Autodesk Inventor part; units mm, degrees
(part 2 of 3)
  spline S225 degree 2 poles (-23.0863, -3.6473) (-22.622, -3.6473) (-22.0662, -4.2796) (-22.0662, -4.8551) knots 0 0 0 1 2 2 2
  spline S226 degree 2 poles (-22.4639, -4.8551) (-22.4639, -4.4105) (-22.7874, -3.9782) (-23.0863, -3.9782) knots 0 0 0 1 2 2 2
  spline S227 degree 2 poles (-23.0863, -3.9782) (-23.3852, -3.9782) (-23.7112, -4.4105) (-23.7112, -4.8551) knots 0 0 0 1 2 2 2
  spline S228 degree 2 poles (-23.7112, -4.8551) (-23.7112, -5.2874) (-23.3852, -5.732) (-23.0863, -5.732) knots 0 0 0 1 2 2 2
  spline S229 degree 2 poles (-23.0863, -5.732) (-22.7899, -5.732) (-22.4639, -5.2948) (-22.4639, -4.8551) knots 0 0 0 1 2 2 2
  line L249 (-1.1, 56.7348) -> (1.5874, 56.7348)
  line L250 (1.5874, 56.7348) -> (1.5874, 57.7574)
  line L251 (1.5874, 57.7574) -> (1.948, 57.7574)
  line L252 (1.948, 57.7574) -> (1.948, 55.3071)
  line L253 (1.948, 55.3071) -> (1.5874, 55.3071)
  line L254 (1.5874, 55.3071) -> (1.5874, 56.3297)
  line L255 (1.5874, 56.3297) -> (-1.1, 56.3297)
  line L256 (-1.1, 56.3297) -> (-1.1, 56.7348)
  spline S230 degree 2 poles (0.0436, 53.1483) (-0.5344, 53.1483) (-1.1642, 53.7041) (-1.1642, 54.1685) knots 0 0 0 1 2 2 2
  spline S231 degree 2 poles (-1.1642, 54.1685) (-1.1642, 54.6452) (-0.5146, 55.191) (0.0436, 55.191) knots 0 0 0 1 2 2 2
  spline S232 degree 2 poles (0.0436, 55.191) (0.6167, 55.191) (1.2515, 54.6279) (1.2515, 54.1685) knots 0 0 0 1 2 2 2
  spline S233 degree 2 poles (1.2515, 54.1685) (1.2515, 53.7041) (0.6191, 53.1483) (0.0436, 53.1483) knots 0 0 0 1 2 2 2
  spline S234 degree 2 poles (0.0436, 53.546) (0.4882, 53.546) (0.9205, 53.8696) (0.9205, 54.1685) knots 0 0 0 1 2 2 2
  spline S235 degree 2 poles (0.9205, 54.1685) (0.9205, 54.4673) (0.4882, 54.7934) (0.0436, 54.7934) knots 0 0 0 1 2 2 2
  spline S236 degree 2 poles (0.0436, 54.7934) (-0.3886, 54.7934) (-0.8332, 54.4673) (-0.8332, 54.1685) knots 0 0 0 1 2 2 2
  spline S237 degree 2 poles (-0.8332, 54.1685) (-0.8332, 53.8721) (-0.396, 53.546) (0.0436, 53.546) knots 0 0 0 1 2 2 2
  line L257 (0.7747, 51.5404) -> (0.7747, 51.5601)
  spline S238 degree 2 poles (0.7747, 51.5601) (0.7871, 51.6046) (0.792, 51.7009) (0.792, 51.7676) knots 0 0 0 1 2 2 2
  spline S239 degree 2 poles (0.792, 51.7676) (0.792, 51.9232) (0.6562, 52.2295) (0.5228, 52.3678) knots 0 0 0 1 2 2 2
  line L258 (0.5228, 52.3678) -> (-1.1, 52.3678)
  line L259 (-1.1, 52.3678) -> (-1.1, 52.7531)
  line L260 (-1.1, 52.7531) -> (1.1872, 52.7531)
  line L261 (1.1872, 52.7531) -> (1.1872, 52.3678)
  line L262 (1.1872, 52.3678) -> (0.8464, 52.3678)
  spline S240 degree 2 poles (0.8464, 52.3678) (1.0341, 52.1579) (1.1872, 51.8442) (1.1872, 51.696) knots 0 0 0 1 2 2 2
  spline S241 degree 2 poles (1.1872, 51.696) (1.1872, 51.6367) (1.1823, 51.5774) (1.1749, 51.5404) knots 0 0 0 1 2 2 2
  line L263 (1.1749, 51.5404) -> (0.7747, 51.5404)
  line L264 (1.948, 47.6921) -> (-1.1, 48.7418)
  line L265 (-1.1, 48.7418) -> (-1.1, 49.179)
  line L266 (-1.1, 49.179) -> (1.948, 50.2288)
  line L267 (1.948, 50.2288) -> (1.948, 49.7941)
  line L268 (1.948, 49.7941) -> (-0.5838, 48.9493)
  line L269 (-0.5838, 48.9493) -> (1.948, 48.1046)
  line L270 (1.948, 48.1046) -> (1.948, 47.6921)
  spline S242 degree 2 poles (-1.1519, 46.4373) (-1.1519, 46.9856) (-0.5368, 47.5883) (0.0313, 47.5883) knots 0 0 0 1 2 2 2
  spline S243 degree 2 poles (0.0313, 47.5883) (0.5895, 47.5883) (1.2515, 47.0029) (1.2515, 46.5312) knots 0 0 0 1 2 2 2
  spline S244 degree 2 poles (1.2515, 46.5312) (1.2515, 46.3187) (1.128, 45.9902) (0.997, 45.8692) knots 0 0 0 1 2 2 2
  spline S245 degree 2 poles (0.997, 45.8692) (0.8661, 45.7457) (0.4882, 45.6148) (0.2141, 45.6148) knots 0 0 0 1 2 2 2
  line L271 (0.2141, 45.6148) -> (0.0041, 45.6148)
  line L272 (0.0041, 45.6148) -> (0.0041, 47.1981)
  spline S246 degree 2 poles (0.0041, 47.1981) (-0.3936, 47.1981) (-0.8159, 46.7979) (-0.8159, 46.4422) knots 0 0 0 1 2 2 2
  spline S247 degree 2 poles (-0.8159, 46.4422) (-0.8159, 46.3163) (-0.7591, 46.0717) (-0.7147, 45.9729) knots 0 0 0 1 2 2 2
  spline S248 degree 2 poles (-0.7147, 45.9729) (-0.6653, 45.8692) (-0.5788, 45.7259) (-0.5393, 45.679) knots 0 0 0 1 2 2 2
  line L273 (-0.5393, 45.679) -> (-0.5393, 45.6568)
  line L274 (-0.5393, 45.6568) -> (-0.9592, 45.6568)
  spline S249 degree 2 poles (-0.9592, 45.6568) (-0.9864, 45.7235) (-1.0654, 45.926) (-1.0876, 46.0051) knots 0 0 0 1 2 2 2
  spline S250 degree 2 poles (-1.0876, 46.0051) (-1.1198, 46.1162) (-1.1519, 46.299) (-1.1519, 46.4373) knots 0 0 0 1 2 2 2
  spline S251 degree 2 poles (0.298, 45.9902) (0.4536, 45.9952) (0.6809, 46.0594) (0.7575, 46.1211) knots 0 0 0 1 2 2 2
  spline S252 degree 2 poles (0.7575, 46.1211) (0.8439, 46.1878) (0.9353, 46.3978) (0.9353, 46.5534) knots 0 0 0 1 2 2 2
  spline S253 degree 2 poles (0.9353, 46.5534) (0.9353, 46.7065) (0.8439, 46.9214) (0.755, 47.0103) knots 0 0 0 1 2 2 2
  spline S254 degree 2 poles (0.755, 47.0103) (0.6636, 47.0968) (0.4438, 47.1857) (0.298, 47.1981) knots 0 0 0 1 2 2 2
  line L275 (0.298, 47.1981) -> (0.298, 45.9902)
  line L276 (0.7747, 44.0117) -> (0.7747, 44.0315)
  spline S255 degree 2 poles (0.7747, 44.0315) (0.7871, 44.076) (0.792, 44.1723) (0.792, 44.239) knots 0 0 0 1 2 2 2
  spline S256 degree 2 poles (0.792, 44.239) (0.792, 44.3946) (0.6562, 44.7009) (0.5228, 44.8392) knots 0 0 0 1 2 2 2
  line L277 (0.5228, 44.8392) -> (-1.1, 44.8392)
  line L278 (-1.1, 44.8392) -> (-1.1, 45.2245)
  line L279 (-1.1, 45.2245) -> (1.1872, 45.2245)
  line L280 (1.1872, 45.2245) -> (1.1872, 44.8392)
  line L281 (1.1872, 44.8392) -> (0.8464, 44.8392)
  spline S257 degree 2 poles (0.8464, 44.8392) (1.0341, 44.6293) (1.1872, 44.3156) (1.1872, 44.1674) knots 0 0 0 1 2 2 2
  spline S258 degree 2 poles (1.1872, 44.1674) (1.1872, 44.1081) (1.1823, 44.0488) (1.1749, 44.0117) knots 0 0 0 1 2 2 2
  line L282 (1.1749, 44.0117) -> (0.7747, 44.0117)
  spline S259 degree 2 poles (-1.4656, 43.6314) (-1.4829, 43.5918) (-1.5372, 43.4412) (-1.5594, 43.3448) knots 0 0 0 1 2 2 2
  spline S260 degree 2 poles (-1.5594, 43.3448) (-1.5866, 43.2386) (-1.6187, 43.0583) (-1.6187, 42.9521) knots 0 0 0 1 2 2 2
  spline S261 degree 2 poles (-1.6187, 42.9521) (-1.6187, 42.7743) (-1.5248, 42.5273) (-1.4409, 42.4581) knots 0 0 0 1 2 2 2
  spline S262 degree 2 poles (-1.4409, 42.4581) (-1.3569, 42.3914) (-1.137, 42.3395) (-0.9963, 42.3395) knots 0 0 0 1 2 2 2
  line L283 (-0.9963, 42.3395) -> (-0.7962, 42.3395)
  spline S263 degree 2 poles (-0.7962, 42.3395) (-0.932, 42.4952) (-1.0605, 42.794) (-1.0605, 43.0188) knots 0 0 0 1 2 2 2
  spline S264 degree 2 poles (-1.0605, 43.0188) (-1.0605, 43.4091) (-0.48, 43.871) (0.0658, 43.871) knots 0 0 0 1 2 2 2
  spline S265 degree 2 poles (0.0658, 43.871) (0.3499, 43.871) (0.7896, 43.7104) (0.9452, 43.577) knots 0 0 0 1 2 2 2
  spline S266 degree 2 poles (0.9452, 43.577) (1.0909, 43.4486) (1.2515, 43.0954) (1.2515, 42.9077) knots 0 0 0 1 2 2 2
  spline S267 degree 2 poles (1.2515, 42.9077) (1.2515, 42.7298) (1.1675, 42.4705) (1.0909, 42.3395) knots 0 0 0 1 2 2 2
  line L284 (1.0909, 42.3395) -> (1.1872, 42.3173)
  line L285 (1.1872, 42.3173) -> (1.1872, 41.9542)
  line L286 (1.1872, 41.9542) -> (-0.8382, 41.9542)
  spline S268 degree 2 poles (-0.8382, 41.9542) (-1.4211, 41.9542) (-1.9645, 42.4606) (-1.9645, 42.9818) knots 0 0 0 1 2 2 2
  spline S269 degree 2 poles (-1.9645, 42.9818) (-1.9645, 43.1497) (-1.9102, 43.5005) (-1.8657, 43.6511) knots 0 0 0 1 2 2 2
  line L287 (-1.8657, 43.6511) -> (-1.4656, 43.6511)
  line L288 (-1.4656, 43.6511) -> (-1.4656, 43.6314)
  line L289 (-0.48, 42.3395) -> (0.7772, 42.3395)
  spline S270 degree 2 poles (0.7772, 42.3395) (0.8464, 42.4828) (0.9057, 42.7249) (0.9057, 42.8459) knots 0 0 0 1 2 2 2
  spline S271 degree 2 poles (0.9057, 42.8459) (0.9057, 43.1374) (0.4759, 43.4733) (0.0733, 43.4733) knots 0 0 0 1 2 2 2
  spline S272 degree 2 poles (0.0733, 43.4733) (-0.3071, 43.4733) (-0.7048, 43.2189) (-0.7048, 42.9324) knots 0 0 0 1 2 2 2
  spline S273 degree 2 poles (-0.7048, 42.9324) (-0.7048, 42.7817) (-0.5862, 42.4655) (-0.48, 42.3395) knots 0 0 0 1 2 2 2
  spline S274 degree 2 poles (-0.8579, 40.1215) (-0.8925, 40.1684) (-1.016, 40.3265) (-1.0531, 40.4006) knots 0 0 0 1 2 2 2
  spline S275 degree 2 poles (-1.0531, 40.4006) (-1.1074, 40.5019) (-1.1642, 40.692) (-1.1642, 40.8649) knots 0 0 0 1 2 2 2
  spline S276 degree 2 poles (-1.1642, 40.8649) (-1.1642, 41.0057) (-1.058, 41.2601) (-0.9617, 41.3565) knots 0 0 0 1 2 2 2
  spline S277 degree 2 poles (-0.9617, 41.3565) (-0.8678, 41.4479) (-0.5912, 41.559) (-0.438, 41.559) knots 0 0 0 1 2 2 2
  spline S278 degree 2 poles (-0.438, 41.559) (-0.2009, 41.559) (0.135, 41.3589) (0.2313, 41.1416) knots 0 0 0 1 2 2 2
  spline S279 degree 2 poles (0.2313, 41.1416) (0.3203, 40.9489) (0.387, 40.4253) (0.4042, 40.1215) knots 0 0 0 1 2 2 2
  line L290 (0.4042, 40.1215) -> (0.4783, 40.1215)
  spline S280 degree 2 poles (0.4783, 40.1215) (0.6117, 40.1215) (0.7772, 40.203) (0.8241, 40.2771) knots 0 0 0 1 2 2 2
  spline S281 degree 2 poles (0.8241, 40.2771) (0.8711, 40.3512) (0.9007, 40.5636) (0.9007, 40.6772) knots 0 0 0 1 2 2 2
  spline S282 degree 2 poles (0.9007, 40.6772) (0.9007, 40.8106) (0.8217, 41.1712) (0.7451, 41.3515) knots 0 0 0 1 2 2 2
  line L291 (0.7451, 41.3515) -> (0.7451, 41.3738)
  line L292 (0.7451, 41.3738) -> (1.1378, 41.3738)
  spline S283 degree 2 poles (1.1378, 41.3738) (1.1675, 41.2676) (1.2416, 40.8699) (1.2416, 40.6748) knots 0 0 0 1 2 2 2
  spline S284 degree 2 poles (1.2416, 40.6748) (1.2416, 40.4376) (1.1675, 40.1141) (1.0711, 39.9856) knots 0 0 0 1 2 2 2
  spline S285 degree 2 poles (1.0711, 39.9856) (0.9773, 39.8596) (0.6784, 39.7361) (0.4635, 39.7361) knots 0 0 0 1 2 2 2
  line L293 (0.4635, 39.7361) -> (-1.1, 39.7361)
  line L294 (-1.1, 39.7361) -> (-1.1, 40.1215)
  line L295 (-1.1, 40.1215) -> (-0.8579, 40.1215)
  line L296 (-0.5368, 40.1215) -> (0.098, 40.1215)
  spline S286 degree 2 poles (0.098, 40.1215) (0.0856, 40.2598) (0.0436, 40.6772) (0.0041, 40.8081) knots 0 0 0 1 2 2 2
  spline S287 degree 2 poles (0.0041, 40.8081) (-0.0428, 40.9613) (-0.238, 41.1613) (-0.4109, 41.1613) knots 0 0 0 1 2 2 2
  spline S288 degree 2 poles (-0.4109, 41.1613) (-0.6085, 41.1613) (-0.8085, 40.939) (-0.8085, 40.7266) knots 0 0 0 1 2 2 2
  spline S289 degree 2 poles (-0.8085, 40.7266) (-0.8085, 40.5463) (-0.6529, 40.2499) (-0.5368, 40.1215) knots 0 0 0 1 2 2 2
  spline S290 degree 2 poles (-1.1445, 38.5036) (-1.1445, 38.8173) (-0.7863, 39.1705) (-0.3985, 39.1705) knots 0 0 0 1 2 2 2
  line L297 (-0.3985, 39.1705) -> (0.8686, 39.1705)
  line L298 (0.8686, 39.1705) -> (0.8686, 39.4299)
  line L299 (0.8686, 39.4299) -> (1.1872, 39.4299)
  line L300 (1.1872, 39.4299) -> (1.1872, 39.1705)
  line L301 (1.1872, 39.1705) -> (1.8443, 39.1705)
  line L302 (1.8443, 39.1705) -> (1.8443, 38.7852)
  line L303 (1.8443, 38.7852) -> (1.1872, 38.7852)
  line L304 (1.1872, 38.7852) -> (1.1872, 38.0763)
  line L305 (1.1872, 38.0763) -> (0.8686, 38.0763)
  line L306 (0.8686, 38.0763) -> (0.8686, 38.7852)
  line L307 (0.8686, 38.7852) -> (-0.2207, 38.7852)
  spline S291 degree 2 poles (-0.2207, 38.7852) (-0.3936, 38.7852) (-0.5838, 38.7728) (-0.6653, 38.7309) knots 0 0 0 1 2 2 2
  spline S292 degree 2 poles (-0.6653, 38.7309) (-0.7369, 38.6963) (-0.8085, 38.5407) (-0.8085, 38.4073) knots 0 0 0 1 2 2 2
  spline S293 degree 2 poles (-0.8085, 38.4073) (-0.8085, 38.3134) (-0.7517, 38.138) (-0.7344, 38.0985) knots 0 0 0 1 2 2 2
  line L308 (-0.7344, 38.0985) -> (-0.7344, 38.0763)
  line L309 (-0.7344, 38.0763) -> (-1.0802, 38.0763)
  spline S294 degree 2 poles (-1.0802, 38.0763) (-1.1099, 38.185) (-1.1445, 38.4073) (-1.1445, 38.5036) knots 0 0 0 1 2 2 2
  spline S295 degree 2 poles (-0.8579, 36.5177) (-0.8925, 36.5646) (-1.016, 36.7227) (-1.0531, 36.7968) knots 0 0 0 1 2 2 2
  spline S296 degree 2 poles (-1.0531, 36.7968) (-1.1074, 36.8981) (-1.1642, 37.0883) (-1.1642, 37.2612) knots 0 0 0 1 2 2 2
  spline S297 degree 2 poles (-1.1642, 37.2612) (-1.1642, 37.402) (-1.058, 37.6564) (-0.9617, 37.7527) knots 0 0 0 1 2 2 2
  spline S298 degree 2 poles (-0.9617, 37.7527) (-0.8678, 37.8441) (-0.5912, 37.9553) (-0.438, 37.9553) knots 0 0 0 1 2 2 2
  spline S299 degree 2 poles (-0.438, 37.9553) (-0.2009, 37.9553) (0.135, 37.7552) (0.2313, 37.5378) knots 0 0 0 1 2 2 2
  spline S300 degree 2 poles (0.2313, 37.5378) (0.3203, 37.3452) (0.387, 36.8215) (0.4042, 36.5177) knots 0 0 0 1 2 2 2
  line L310 (0.4042, 36.5177) -> (0.4783, 36.5177)
  spline S301 degree 2 poles (0.4783, 36.5177) (0.6117, 36.5177) (0.7772, 36.5992) (0.8241, 36.6733) knots 0 0 0 1 2 2 2
  spline S302 degree 2 poles (0.8241, 36.6733) (0.8711, 36.7474) (0.9007, 36.9599) (0.9007, 37.0735) knots 0 0 0 1 2 2 2
  spline S303 degree 2 poles (0.9007, 37.0735) (0.9007, 37.2069) (0.8217, 37.5675) (0.7451, 37.7478) knots 0 0 0 1 2 2 2
  line L311 (0.7451, 37.7478) -> (0.7451, 37.77)
  line L312 (0.7451, 37.77) -> (1.1378, 37.77)
  spline S304 degree 2 poles (1.1378, 37.77) (1.1675, 37.6638) (1.2416, 37.2661) (1.2416, 37.071) knots 0 0 0 1 2 2 2
  spline S305 degree 2 poles (1.2416, 37.071) (1.2416, 36.8339) (1.1675, 36.5103) (1.0711, 36.3819) knots 0 0 0 1 2 2 2
  spline S306 degree 2 poles (1.0711, 36.3819) (0.9773, 36.2559) (0.6784, 36.1324) (0.4635, 36.1324) knots 0 0 0 1 2 2 2
  line L313 (0.4635, 36.1324) -> (-1.1, 36.1324)
  line L314 (-1.1, 36.1324) -> (-1.1, 36.5177)
  line L315 (-1.1, 36.5177) -> (-0.8579, 36.5177)
  line L316 (-0.5368, 36.5177) -> (0.098, 36.5177)
  spline S307 degree 2 poles (0.098, 36.5177) (0.0856, 36.656) (0.0436, 37.0735) (0.0041, 37.2044) knots 0 0 0 1 2 2 2
  spline S308 degree 2 poles (0.0041, 37.2044) (-0.0428, 37.3575) (-0.238, 37.5576) (-0.4109, 37.5576) knots 0 0 0 1 2 2 2
  spline S309 degree 2 poles (-0.4109, 37.5576) (-0.6085, 37.5576) (-0.8085, 37.3353) (-0.8085, 37.1229) knots 0 0 0 1 2 2 2
  spline S310 degree 2 poles (-0.8085, 37.1229) (-0.8085, 36.9426) (-0.6529, 36.6462) (-0.5368, 36.5177) knots 0 0 0 1 2 2 2
  spline S311 degree 2 poles (28.9328, 4.0036) (28.6019, 4.0036) (28.1375, 4.1419) (27.9325, 4.2407) knots 0 0 0 1 2 2 2
  line L317 (27.9325, 4.2407) -> (27.9325, 4.7495)
  line L318 (27.9325, 4.7495) -> (27.9621, 4.7495)
  spline S312 degree 2 poles (27.9621, 4.7495) (28.1622, 4.5618) (28.6686, 4.3543) (28.9032, 4.3543) knots 0 0 0 1 2 2 2
  spline S313 degree 2 poles (28.9032, 4.3543) (29.2391, 4.3543) (29.5825, 4.6335) (29.5825, 4.8632) knots 0 0 0 1 2 2 2
  spline S314 degree 2 poles (29.5825, 4.8632) (29.5825, 5.046) (29.4022, 5.2732) (29.207, 5.33) knots 0 0 0 1 2 2 2
  spline S315 degree 2 poles (29.207, 5.33) (29.0662, 5.3695) (28.8316, 5.4239) (28.6562, 5.4683) knots 0 0 0 1 2 2 2
  spline S316 degree 2 poles (28.6562, 5.4683) (28.4981, 5.5103) (28.2487, 5.6363) (28.1523, 5.7376) knots 0 0 0 1 2 2 2
  spline S317 degree 2 poles (28.1523, 5.7376) (28.0585, 5.8388) (27.9547, 6.1105) (27.9547, 6.2884) knots 0 0 0 1 2 2 2
  spline S318 degree 2 poles (27.9547, 6.2884) (27.9547, 6.6589) (28.5327, 7.1603) (28.9798, 7.1603) knots 0 0 0 1 2 2 2
  spline S319 degree 2 poles (28.9798, 7.1603) (29.2367, 7.1603) (29.6911, 7.059) (29.8863, 6.9627) knots 0 0 0 1 2 2 2
  line L319 (29.8863, 6.9627) -> (29.8863, 6.4786)
  line L320 (29.8863, 6.4786) -> (29.8566, 6.4786)
  spline S320 degree 2 poles (29.8566, 6.4786) (29.7109, 6.6119) (29.2564, 6.8095) (29.0069, 6.8095) knots 0 0 0 1 2 2 2
  spline S321 degree 2 poles (29.0069, 6.8095) (28.7254, 6.8095) (28.3771, 6.5453) (28.3771, 6.3304) knots 0 0 0 1 2 2 2
  spline S322 degree 2 poles (28.3771, 6.3304) (28.3771, 6.1377) (28.5821, 5.908) (28.7748, 5.8561) knots 0 0 0 1 2 2 2
  spline S323 degree 2 poles (28.7748, 5.8561) (28.9032, 5.8215) (29.2762, 5.7326) (29.3997, 5.6956) knots 0 0 0 1 2 2 2
  spline S324 degree 2 poles (29.3997, 5.6956) (29.7134, 5.5992) (30.0048, 5.2114) (30.0048, 4.9274) knots 0 0 0 1 2 2 2
  spline S325 degree 2 poles (30.0048, 4.9274) (30.0048, 4.7471) (29.8591, 4.4013) (29.7282, 4.2802) knots 0 0 0 1 2 2 2
  spline S326 degree 2 poles (29.7282, 4.2802) (29.5825, 4.1469) (29.212, 4.0036) (28.9328, 4.0036) knots 0 0 0 1 2 2 2
  spline S327 degree 2 poles (32.2674, 5.2016) (32.2674, 4.6236) (31.7116, 3.9937) (31.2473, 3.9937) knots 0 0 0 1 2 2 2
  spline S328 degree 2 poles (31.2473, 3.9937) (30.7705, 3.9937) (30.2247, 4.6433) (30.2247, 5.2016) knots 0 0 0 1 2 2 2
  spline S329 degree 2 poles (30.2247, 5.2016) (30.2247, 5.7746) (30.7878, 6.4094) (31.2473, 6.4094) knots 0 0 0 1 2 2 2
  spline S330 degree 2 poles (31.2473, 6.4094) (31.7116, 6.4094) (32.2674, 5.7771) (32.2674, 5.2016) knots 0 0 0 1 2 2 2
  spline S331 degree 2 poles (31.8697, 5.2016) (31.8697, 5.6462) (31.5461, 6.0784) (31.2473, 6.0784) knots 0 0 0 1 2 2 2
  spline S332 degree 2 poles (31.2473, 6.0784) (30.9484, 6.0784) (30.6223, 5.6462) (30.6223, 5.2016) knots 0 0 0 1 2 2 2
  spline S333 degree 2 poles (30.6223, 5.2016) (30.6223, 4.7693) (30.9484, 4.3247) (31.2473, 4.3247) knots 0 0 0 1 2 2 2
  spline S334 degree 2 poles (31.2473, 4.3247) (31.5437, 4.3247) (31.8697, 4.7619) (31.8697, 5.2016) knots 0 0 0 1 2 2 2
  spline S335 degree 2 poles (33.5715, 4.0061) (33.3344, 4.0061) (32.9417, 4.1518) (32.8009, 4.3) knots 0 0 0 1 2 2 2
  spline S336 degree 2 poles (32.8009, 4.3) (32.6601, 4.4457) (32.5045, 4.8953) (32.5045, 5.1966) knots 0 0 0 1 2 2 2
  spline S337 degree 2 poles (32.5045, 5.1966) (32.5045, 5.498) (32.665, 5.9376) (32.8009, 6.0858) knots 0 0 0 1 2 2 2
  spline S338 degree 2 poles (32.8009, 6.0858) (32.9367, 6.2365) (33.3394, 6.397) (33.5715, 6.397) knots 0 0 0 1 2 2 2
  spline S339 degree 2 poles (33.5715, 6.397) (33.7593, 6.397) (34.11, 6.2908) (34.2459, 6.2217) knots 0 0 0 1 2 2 2
  line L321 (34.2459, 6.2217) -> (34.2459, 5.7894)
  line L322 (34.2459, 5.7894) -> (34.2236, 5.7894)
  spline S340 degree 2 poles (34.2236, 5.7894) (34.1816, 5.824) (34.0532, 5.9129) (33.9618, 5.9599) knots 0 0 0 1 2 2 2
  spline S341 degree 2 poles (33.9618, 5.9599) (33.8803, 5.9994) (33.6629, 6.0611) (33.5641, 6.0611) knots 0 0 0 1 2 2 2
  spline S342 degree 2 poles (33.5641, 6.0611) (33.2653, 6.0611) (32.9022, 5.6091) (32.9022, 5.1966) knots 0 0 0 1 2 2 2
  spline S343 degree 2 poles (32.9022, 5.1966) (32.9022, 4.794) (33.2529, 4.342) (33.5641, 4.342) knots 0 0 0 1 2 2 2
  spline S344 degree 2 poles (33.5641, 4.342) (33.7519, 4.342) (34.0927, 4.4976) (34.2236, 4.6186) knots 0 0 0 1 2 2 2
  line L323 (34.2236, 4.6186) -> (34.2459, 4.6186)
  line L324 (34.2459, 4.6186) -> (34.2459, 4.1864)
  spline S345 degree 2 poles (34.2459, 4.1864) (34.189, 4.1592) (34.0161, 4.0826) (33.947, 4.0654) knots 0 0 0 1 2 2 2
  spline S346 degree 2 poles (33.947, 4.0654) (33.8482, 4.0357) (33.6926, 4.0061) (33.5715, 4.0061) knots 0 0 0 1 2 2 2
  spline S347 degree 2 poles (35.5056, 4.0061) (35.2684, 4.0061) (34.8757, 4.1518) (34.7349, 4.3) knots 0 0 0 1 2 2 2
  spline S348 degree 2 poles (34.7349, 4.3) (34.5941, 4.4457) (34.4385, 4.8953) (34.4385, 5.1966) knots 0 0 0 1 2 2 2
  spline S349 degree 2 poles (34.4385, 5.1966) (34.4385, 5.498) (34.5991, 5.9376) (34.7349, 6.0858) knots 0 0 0 1 2 2 2
  spline S350 degree 2 poles (34.7349, 6.0858) (34.8708, 6.2365) (35.2734, 6.397) (35.5056, 6.397) knots 0 0 0 1 2 2 2
  spline S351 degree 2 poles (35.5056, 6.397) (35.6933, 6.397) (36.044, 6.2908) (36.1799, 6.2217) knots 0 0 0 1 2 2 2
  line L325 (36.1799, 6.2217) -> (36.1799, 5.7894)
  line L326 (36.1799, 5.7894) -> (36.1576, 5.7894)
  spline S352 degree 2 poles (36.1576, 5.7894) (36.1157, 5.824) (35.9872, 5.9129) (35.8958, 5.9599) knots 0 0 0 1 2 2 2
  spline S353 degree 2 poles (35.8958, 5.9599) (35.8143, 5.9994) (35.597, 6.0611) (35.4982, 6.0611) knots 0 0 0 1 2 2 2
  spline S354 degree 2 poles (35.4982, 6.0611) (35.1993, 6.0611) (34.8362, 5.6091) (34.8362, 5.1966) knots 0 0 0 1 2 2 2
  spline S355 degree 2 poles (34.8362, 5.1966) (34.8362, 4.794) (35.1869, 4.342) (35.4982, 4.342) knots 0 0 0 1 2 2 2
  spline S356 degree 2 poles (35.4982, 4.342) (35.6859, 4.342) (36.0267, 4.4976) (36.1576, 4.6186) knots 0 0 0 1 2 2 2
  line L327 (36.1576, 4.6186) -> (36.1799, 4.6186)
  line L328 (36.1799, 4.6186) -> (36.1799, 4.1864)
  spline S357 degree 2 poles (36.1799, 4.1864) (36.1231, 4.1592) (35.9502, 4.0826) (35.881, 4.0654) knots 0 0 0 1 2 2 2
  spline S358 degree 2 poles (35.881, 4.0654) (35.7822, 4.0357) (35.6266, 4.0061) (35.5056, 4.0061) knots 0 0 0 1 2 2 2
  line L329 (36.9234, 4.0579) -> (36.538, 4.0579)
  line L330 (36.538, 4.0579) -> (36.538, 6.3452)
  line L331 (36.538, 6.3452) -> (36.9234, 6.3452)
  line L332 (36.9234, 6.3452) -> (36.9234, 4.0579)
  line L333 (36.9505, 6.7256) -> (36.5133, 6.7256)
  line L334 (36.5133, 6.7256) -> (36.5133, 7.1257)
  line L335 (36.5133, 7.1257) -> (36.9505, 7.1257)
  line L336 (36.9505, 7.1257) -> (36.9505, 6.7256)
  spline S359 degree 2 poles (39.3687, 5.2016) (39.3687, 4.6236) (38.8129, 3.9937) (38.3486, 3.9937) knots 0 0 0 1 2 2 2
  spline S360 degree 2 poles (38.3486, 3.9937) (37.8718, 3.9937) (37.326, 4.6433) (37.326, 5.2016) knots 0 0 0 1 2 2 2
  spline S361 degree 2 poles (37.326, 5.2016) (37.326, 5.7746) (37.8891, 6.4094) (38.3486, 6.4094) knots 0 0 0 1 2 2 2
  spline S362 degree 2 poles (38.3486, 6.4094) (38.8129, 6.4094) (39.3687, 5.7771) (39.3687, 5.2016) knots 0 0 0 1 2 2 2
  spline S363 degree 2 poles (38.971, 5.2016) (38.971, 5.6462) (38.6474, 6.0784) (38.3486, 6.0784) knots 0 0 0 1 2 2 2
  spline S364 degree 2 poles (38.3486, 6.0784) (38.0497, 6.0784) (37.7236, 5.6462) (37.7236, 5.2016) knots 0 0 0 1 2 2 2
  spline S365 degree 2 poles (37.7236, 5.2016) (37.7236, 4.7693) (38.0497, 4.3247) (38.3486, 4.3247) knots 0 0 0 1 2 2 2
  spline S366 degree 2 poles (38.3486, 4.3247) (38.645, 4.3247) (38.971, 4.7619) (38.971, 5.2016) knots 0 0 0 1 2 2 2
  line L337 (42.8687, 4.0579) -> (41.1026, 4.0579)
  line L338 (41.1026, 4.0579) -> (41.1026, 7.1059)
  line L339 (41.1026, 7.1059) -> (41.5077, 7.1059)
  line L340 (41.5077, 7.1059) -> (41.5077, 4.4186)
  line L341 (41.5077, 4.4186) -> (42.8687, 4.4186)
  line L342 (42.8687, 4.4186) -> (42.8687, 4.0579)
  spline S367 degree 2 poles (44.1506, 4.0061) (43.6023, 4.0061) (42.9996, 4.6211) (42.9996, 5.1892) knots 0 0 0 1 2 2 2
  spline S368 degree 2 poles (42.9996, 5.1892) (42.9996, 5.7474) (43.585, 6.4094) (44.0568, 6.4094) knots 0 0 0 1 2 2 2
  spline S369 degree 2 poles (44.0568, 6.4094) (44.2692, 6.4094) (44.5977, 6.2859) (44.7187, 6.155) knots 0 0 0 1 2 2 2
  spline S370 degree 2 poles (44.7187, 6.155) (44.8422, 6.0241) (44.9731, 5.6462) (44.9731, 5.372) knots 0 0 0 1 2 2 2
  line L343 (44.9731, 5.372) -> (44.9731, 5.162)
  line L344 (44.9731, 5.162) -> (43.3899, 5.162)
  spline S371 degree 2 poles (43.3899, 5.162) (43.3899, 4.7644) (43.79, 4.342) (44.1457, 4.342) knots 0 0 0 1 2 2 2
  spline S372 degree 2 poles (44.1457, 4.342) (44.2716, 4.342) (44.5162, 4.3988) (44.615, 4.4433) knots 0 0 0 1 2 2 2
  spline S373 degree 2 poles (44.615, 4.4433) (44.7187, 4.4927) (44.862, 4.5791) (44.9089, 4.6186) knots 0 0 0 1 2 2 2
  line L345 (44.9089, 4.6186) -> (44.9311, 4.6186)
  line L346 (44.9311, 4.6186) -> (44.9311, 4.1987)
  spline S374 degree 2 poles (44.9311, 4.1987) (44.8645, 4.1716) (44.6619, 4.0925) (44.5829, 4.0703) knots 0 0 0 1 2 2 2
  spline S375 degree 2 poles (44.5829, 4.0703) (44.4717, 4.0382) (44.2889, 4.0061) (44.1506, 4.0061) knots 0 0 0 1 2 2 2
  spline S376 degree 2 poles (44.5977, 5.456) (44.5928, 5.6116) (44.5285, 5.8388) (44.4668, 5.9154) knots 0 0 0 1 2 2 2
  spline S377 degree 2 poles (44.4668, 5.9154) (44.4001, 6.0018) (44.1901, 6.0932) (44.0345, 6.0932) knots 0 0 0 1 2 2 2
  spline S378 degree 2 poles (44.0345, 6.0932) (43.8814, 6.0932) (43.6665, 6.0018) (43.5776, 5.9129) knots 0 0 0 1 2 2 2
  spline S379 degree 2 poles (43.5776, 5.9129) (43.4911, 5.8215) (43.4022, 5.6017) (43.3899, 5.456) knots 0 0 0 1 2 2 2
  line L347 (43.3899, 5.456) -> (44.5977, 5.456)
  spline S380 degree 2 poles (47.2431, 5.2016) (47.2431, 4.6236) (46.6873, 3.9937) (46.223, 3.9937) knots 0 0 0 1 2 2 2
  spline S381 degree 2 poles (46.223, 3.9937) (45.7462, 3.9937) (45.2004, 4.6433) (45.2004, 5.2016) knots 0 0 0 1 2 2 2
  spline S382 degree 2 poles (45.2004, 5.2016) (45.2004, 5.7746) (45.7635, 6.4094) (46.223, 6.4094) knots 0 0 0 1 2 2 2
  spline S383 degree 2 poles (46.223, 6.4094) (46.6873, 6.4094) (47.2431, 5.7771) (47.2431, 5.2016) knots 0 0 0 1 2 2 2
  spline S384 degree 2 poles (46.8454, 5.2016) (46.8454, 5.6462) (46.5218, 6.0784) (46.223, 6.0784) knots 0 0 0 1 2 2 2
  spline S385 degree 2 poles (46.223, 6.0784) (45.9241, 6.0784) (45.598, 5.6462) (45.598, 5.2016) knots 0 0 0 1 2 2 2
  spline S386 degree 2 poles (45.598, 5.2016) (45.598, 4.7693) (45.9241, 4.3247) (46.223, 4.3247) knots 0 0 0 1 2 2 2
  spline S387 degree 2 poles (46.223, 4.3247) (46.5194, 4.3247) (46.8454, 4.7619) (46.8454, 5.2016) knots 0 0 0 1 2 2 2
  line L348 (49.434, 4.0579) -> (49.0487, 4.0579)
  line L349 (49.0487, 4.0579) -> (49.0487, 5.3621)
  spline S388 degree 2 poles (49.0487, 5.3621) (49.0487, 5.5202) (49.019, 5.7919) (48.9746, 5.8734) knots 0 0 0 1 2 2 2
  spline S389 degree 2 poles (48.9746, 5.8734) (48.9276, 5.9599) (48.7597, 6.0438) (48.6164, 6.0438) knots 0 0 0 1 2 2 2
  spline S390 degree 2 poles (48.6164, 6.0438) (48.4731, 6.0438) (48.1693, 5.8907) (48.0236, 5.7672) knots 0 0 0 1 2 2 2
  line L350 (48.0236, 5.7672) -> (48.0236, 4.0579)
  line L351 (48.0236, 4.0579) -> (47.6383, 4.0579)
  line L352 (47.6383, 4.0579) -> (47.6383, 6.3452)
  line L353 (47.6383, 6.3452) -> (48.0236, 6.3452)
  line L354 (48.0236, 6.3452) -> (48.0236, 6.0908)
  spline S391 degree 2 poles (48.0236, 6.0908) (48.1965, 6.2464) (48.53, 6.4094) (48.7177, 6.4094) knots 0 0 0 1 2 2 2
  spline S392 degree 2 poles (48.7177, 6.4094) (49.0536, 6.4094) (49.434, 5.9648) (49.434, 5.5424) knots 0 0 0 1 2 2 2
  line L355 (49.434, 5.5424) -> (49.434, 4.0579)
  spline S393 degree 2 poles (51.2494, 4.3) (51.2025, 4.2654) (51.0444, 4.1419) (50.9703, 4.1049) knots 0 0 0 1 2 2 2
  spline S394 degree 2 poles (50.9703, 4.1049) (50.8691, 4.0505) (50.6789, 3.9937) (50.506, 3.9937) knots 0 0 0 1 2 2 2
  spline S395 degree 2 poles (50.506, 3.9937) (50.3652, 3.9937) (50.1108, 4.0999) (50.0144, 4.1963) knots 0 0 0 1 2 2 2
  spline S396 degree 2 poles (50.0144, 4.1963) (49.923, 4.2901) (49.8119, 4.5668) (49.8119, 4.7199) knots 0 0 0 1 2 2 2
  spline S397 degree 2 poles (49.8119, 4.7199) (49.8119, 4.957) (50.012, 5.293) (50.2293, 5.3893) knots 0 0 0 1 2 2 2
  spline S398 degree 2 poles (50.2293, 5.3893) (50.422, 5.4782) (50.9456, 5.5449) (51.2494, 5.5622) knots 0 0 0 1 2 2 2
  line L356 (51.2494, 5.5622) -> (51.2494, 5.6363)
  spline S399 degree 2 poles (51.2494, 5.6363) (51.2494, 5.7697) (51.1679, 5.9352) (51.0938, 5.9821) knots 0 0 0 1 2 2 2
  spline S400 degree 2 poles (51.0938, 5.9821) (51.0197, 6.029) (50.8073, 6.0587) (50.6937, 6.0587) knots 0 0 0 1 2 2 2
  spline S401 degree 2 poles (50.6937, 6.0587) (50.5603, 6.0587) (50.1997, 5.9796) (50.0194, 5.903) knots 0 0 0 1 2 2 2
  line L357 (50.0194, 5.903) -> (49.9971, 5.903)
  line L358 (49.9971, 5.903) -> (49.9971, 6.2958)
  spline S402 degree 2 poles (49.9971, 6.2958) (50.1034, 6.3254) (50.501, 6.3995) (50.6962, 6.3995) knots 0 0 0 1 2 2 2
  spline S403 degree 2 poles (50.6962, 6.3995) (50.9333, 6.3995) (51.2569, 6.3254) (51.3853, 6.2291) knots 0 0 0 1 2 2 2
  spline S404 degree 2 poles (51.3853, 6.2291) (51.5113, 6.1352) (51.6348, 5.8364) (51.6348, 5.6215) knots 0 0 0 1 2 2 2
  line L359 (51.6348, 5.6215) -> (51.6348, 4.0579)
  line L360 (51.6348, 4.0579) -> (51.2494, 4.0579)
  line L361 (51.2494, 4.0579) -> (51.2494, 4.3)
  line L362 (51.2494, 4.6211) -> (51.2494, 5.2559)
  spline S405 degree 2 poles (51.2494, 5.2559) (51.1111, 5.2436) (50.6937, 5.2016) (50.5628, 5.162) knots 0 0 0 1 2 2 2
  spline S406 degree 2 poles (50.5628, 5.162) (50.4096, 5.1151) (50.2096, 4.92) (50.2096, 4.7471) knots 0 0 0 1 2 2 2
  spline S407 degree 2 poles (50.2096, 4.7471) (50.2096, 4.5495) (50.4319, 4.3494) (50.6443, 4.3494) knots 0 0 0 1 2 2 2
  spline S408 degree 2 poles (50.6443, 4.3494) (50.8246, 4.3494) (51.121, 4.505) (51.2494, 4.6211) knots 0 0 0 1 2 2 2
  line L363 (53.3885, 5.9327) -> (53.3687, 5.9327)
  spline S409 degree 2 poles (53.3687, 5.9327) (53.3243, 5.945) (53.2279, 5.95) (53.1612, 5.95) knots 0 0 0 1 2 2 2
  spline S410 degree 2 poles (53.1612, 5.95) (53.0056, 5.95) (52.6993, 5.8141) (52.561, 5.6807) knots 0 0 0 1 2 2 2
  line L364 (52.561, 5.6807) -> (52.561, 4.0579)
  line L365 (52.561, 4.0579) -> (52.1757, 4.0579)
  line L366 (52.1757, 4.0579) -> (52.1757, 6.3452)
  line L367 (52.1757, 6.3452) -> (52.561, 6.3452)
  line L368 (52.561, 6.3452) -> (52.561, 6.0043)
  spline S411 degree 2 poles (52.561, 6.0043) (52.771, 6.192) (53.0847, 6.3452) (53.2329, 6.3452) knots 0 0 0 1 2 2 2
  spline S412 degree 2 poles (53.2329, 6.3452) (53.2921, 6.3452) (53.3514, 6.3402) (53.3885, 6.3328) knots 0 0 0 1 2 2 2
  line L369 (53.3885, 6.3328) -> (53.3885, 5.9327)
  line L370 (55.446, 4.0579) -> (55.0607, 4.0579)
  line L371 (55.0607, 4.0579) -> (55.0607, 4.2901)
  spline S413 degree 2 poles (55.0607, 4.2901) (54.9718, 4.216) (54.8408, 4.1172) (54.7519, 4.0752) knots 0 0 0 1 2 2 2
  spline S414 degree 2 poles (54.7519, 4.0752) (54.6704, 4.0357) (54.495, 3.9937) (54.379, 3.9937) knots 0 0 0 1 2 2 2
  spline S415 degree 2 poles (54.379, 3.9937) (54.1912, 3.9937) (53.8751, 4.1493) (53.7639, 4.3) knots 0 0 0 1 2 2 2
  spline S416 degree 2 poles (53.7639, 4.3) (53.6528, 4.4507) (53.5293, 4.8953) (53.5293, 5.1843) knots 0 0 0 1 2 2 2
  spline S417 degree 2 poles (53.5293, 5.1843) (53.5293, 5.4856) (53.6849, 5.9253) (53.8207, 6.0908) knots 0 0 0 1 2 2 2
  spline S418 degree 2 poles (53.8207, 6.0908) (53.9467, 6.239) (54.2999, 6.4094) (54.495, 6.4094) knots 0 0 0 1 2 2 2
  spline S419 degree 2 poles (54.495, 6.4094) (54.6655, 6.4094) (54.9199, 6.3328) (55.0607, 6.2538) knots 0 0 0 1 2 2 2
  line L372 (55.0607, 6.2538) -> (55.0607, 7.2418)
  line L373 (55.0607, 7.2418) -> (55.446, 7.2418)
  line L374 (55.446, 7.2418) -> (55.446, 4.0579)
  line L375 (55.0607, 4.6137) -> (55.0607, 5.9352)
  spline S420 degree 2 poles (55.0607, 5.9352) (54.9174, 6.0043) (54.6902, 6.0562) (54.5593, 6.0562) knots 0 0 0 1 2 2 2
  spline S421 degree 2 poles (54.5593, 6.0562) (54.2629, 6.0562) (53.9269, 5.6116) (53.9269, 5.1917) knots 0 0 0 1 2 2 2
  spline S422 degree 2 poles (53.9269, 5.1917) (53.9269, 4.7866) (54.1838, 4.3593) (54.4679, 4.3593) knots 0 0 0 1 2 2 2
  spline S423 degree 2 poles (54.4679, 4.3593) (54.6185, 4.3593) (54.9248, 4.4976) (55.0607, 4.6137) knots 0 0 0 1 2 2 2
  spline S424 degree 2 poles (57.8839, 5.2016) (57.8839, 4.6236) (57.3282, 3.9937) (56.8638, 3.9937) knots 0 0 0 1 2 2 2
  spline S425 degree 2 poles (56.8638, 3.9937) (56.3871, 3.9937) (55.8412, 4.6433) (55.8412, 5.2016) knots 0 0 0 1 2 2 2
  spline S426 degree 2 poles (55.8412, 5.2016) (55.8412, 5.7746) (56.4044, 6.4094) (56.8638, 6.4094) knots 0 0 0 1 2 2 2
  spline S427 degree 2 poles (56.8638, 6.4094) (57.3282, 6.4094) (57.8839, 5.7771) (57.8839, 5.2016) knots 0 0 0 1 2 2 2
  spline S428 degree 2 poles (57.4862, 5.2016) (57.4862, 5.6462) (57.1627, 6.0784) (56.8638, 6.0784) knots 0 0 0 1 2 2 2
  spline S429 degree 2 poles (56.8638, 6.0784) (56.5649, 6.0784) (56.2389, 5.6462) (56.2389, 5.2016) knots 0 0 0 1 2 2 2
  spline S430 degree 2 poles (56.2389, 5.2016) (56.2389, 4.7693) (56.5649, 4.3247) (56.8638, 4.3247) knots 0 0 0 1 2 2 2
  spline S431 degree 2 poles (56.8638, 4.3247) (57.1602, 4.3247) (57.4862, 4.7619) (57.4862, 5.2016) knots 0 0 0 1 2 2 2
  line L376 (36.8295, -2.931) -> (35.7797, -5.979)
  line L377 (35.7797, -5.979) -> (35.3425, -5.979)
  line L378 (35.3425, -5.979) -> (34.2928, -2.931)
  line L379 (34.2928, -2.931) -> (34.7275, -2.931)
  line L380 (34.7275, -2.931) -> (35.5723, -5.4627)
  line L381 (35.5723, -5.4627) -> (36.417, -2.931)
  line L382 (36.417, -2.931) -> (36.8295, -2.931)
  line L383 (37.484, -5.979) -> (37.0987, -5.979)
  line L384 (37.0987, -5.979) -> (37.0987, -3.6917)
  line L385 (37.0987, -3.6917) -> (37.484, -3.6917)
  line L386 (37.484, -3.6917) -> (37.484, -5.979)
  line L387 (37.5112, -3.3113) -> (37.074, -3.3113)
  line L388 (37.074, -3.3113) -> (37.074, -2.9112)
  line L389 (37.074, -2.9112) -> (37.5112, -2.9112)
  line L390 (37.5112, -2.9112) -> (37.5112, -3.3113)
  spline S432 degree 2 poles (38.7413, -6.0234) (38.4276, -6.0234) (38.0744, -5.6653) (38.0744, -5.2775) knots 0 0 0 1 2 2 2
  line L391 (38.0744, -5.2775) -> (38.0744, -4.0104)
  line L392 (38.0744, -4.0104) -> (37.815, -4.0104)
  line L393 (37.815, -4.0104) -> (37.815, -3.6917)
  line L394 (37.815, -3.6917) -> (38.0744, -3.6917)
  line L395 (38.0744, -3.6917) -> (38.0744, -3.0347)
  line L396 (38.0744, -3.0347) -> (38.4597, -3.0347)
  line L397 (38.4597, -3.0347) -> (38.4597, -3.6917)
  line L398 (38.4597, -3.6917) -> (39.1686, -3.6917)
  line L399 (39.1686, -3.6917) -> (39.1686, -4.0104)
  line L400 (39.1686, -4.0104) -> (38.4597, -4.0104)
  line L401 (38.4597, -4.0104) -> (38.4597, -5.0996)
  spline S433 degree 2 poles (38.4597, -5.0996) (38.4597, -5.2725) (38.4721, -5.4627) (38.514, -5.5442) knots 0 0 0 1 2 2 2
  spline S434 degree 2 poles (38.514, -5.5442) (38.5486, -5.6159) (38.7042, -5.6875) (38.8376, -5.6875) knots 0 0 0 1 2 2 2
  spline S435 degree 2 poles (38.8376, -5.6875) (38.9315, -5.6875) (39.1068, -5.6307) (39.1464, -5.6134) knots 0 0 0 1 2 2 2
  line L402 (39.1464, -5.6134) -> (39.1686, -5.6134)
  line L403 (39.1686, -5.6134) -> (39.1686, -5.9592)
  spline S436 degree 2 poles (39.1686, -5.9592) (39.0599, -5.9888) (38.8376, -6.0234) (38.7413, -6.0234) knots 0 0 0 1 2 2 2
  spline S437 degree 2 poles (40.1443, -6.0234) (39.8306, -6.0234) (39.4773, -5.6653) (39.4773, -5.2775) knots 0 0 0 1 2 2 2
  line L404 (39.4773, -5.2775) -> (39.4773, -4.0104)
  line L405 (39.4773, -4.0104) -> (39.218, -4.0104)
  line L406 (39.218, -4.0104) -> (39.218, -3.6917)
  line L407 (39.218, -3.6917) -> (39.4773, -3.6917)
  line L408 (39.4773, -3.6917) -> (39.4773, -3.0347)
  line L409 (39.4773, -3.0347) -> (39.8627, -3.0347)
  line L410 (39.8627, -3.0347) -> (39.8627, -3.6917)
  line L411 (39.8627, -3.6917) -> (40.5716, -3.6917)
  line L412 (40.5716, -3.6917) -> (40.5716, -4.0104)
  line L413 (40.5716, -4.0104) -> (39.8627, -4.0104)
  line L414 (39.8627, -4.0104) -> (39.8627, -5.0996)
  spline S438 degree 2 poles (39.8627, -5.0996) (39.8627, -5.2725) (39.875, -5.4627) (39.917, -5.5442) knots 0 0 0 1 2 2 2
  spline S439 degree 2 poles (39.917, -5.5442) (39.9516, -5.6159) (40.1072, -5.6875) (40.2406, -5.6875) knots 0 0 0 1 2 2 2
  spline S440 degree 2 poles (40.2406, -5.6875) (40.3344, -5.6875) (40.5098, -5.6307) (40.5493, -5.6134) knots 0 0 0 1 2 2 2
  line L415 (40.5493, -5.6134) -> (40.5716, -5.6134)
  line L416 (40.5716, -5.6134) -> (40.5716, -5.9592)
  spline S441 degree 2 poles (40.5716, -5.9592) (40.4629, -5.9888) (40.2406, -6.0234) (40.1443, -6.0234) knots 0 0 0 1 2 2 2
  line L417 (41.2483, -5.979) -> (40.863, -5.979)
  line L418 (40.863, -5.979) -> (40.863, -3.6917)
  line L419 (40.863, -3.6917) -> (41.2483, -3.6917)
  line L420 (41.2483, -3.6917) -> (41.2483, -5.979)
  line L421 (41.2755, -3.3113) -> (40.8383, -3.3113)
  line L422 (40.8383, -3.3113) -> (40.8383, -2.9112)
  line L423 (40.8383, -2.9112) -> (41.2755, -2.9112)
  line L424 (41.2755, -2.9112) -> (41.2755, -3.3113)
  spline S442 degree 2 poles (44.4297, -6.0382) (44.1062, -6.0382) (43.5702, -5.8406) (43.3775, -5.6406) knots 0 0 0 1 2 2 2
  spline S443 degree 2 poles (43.3775, -5.6406) (43.1848, -5.438) (42.9798, -4.8403) (42.9798, -4.4525) knots 0 0 0 1 2 2 2
  spline S444 degree 2 poles (42.9798, -4.4525) (42.9798, -4.0845) (43.1873, -3.5015) (43.38, -3.2941) knots 0 0 0 1 2 2 2
  spline S445 degree 2 poles (43.38, -3.2941) (43.5652, -3.094) (44.1086, -2.8766) (44.4322, -2.8766) knots 0 0 0 1 2 2 2
  spline S446 degree 2 poles (44.4322, -2.8766) (44.5878, -2.8766) (44.8694, -2.9211) (44.9978, -2.9606) knots 0 0 0 1 2 2 2
  spline S447 degree 2 poles (44.9978, -2.9606) (45.1016, -2.9902) (45.3535, -3.0989) (45.4301, -3.1384) knots 0 0 0 1 2 2 2
  line L425 (45.4301, -3.1384) -> (45.4301, -3.6275)
  line L426 (45.4301, -3.6275) -> (45.3955, -3.6275)
  spline S448 degree 2 poles (45.3955, -3.6275) (45.3189, -3.5608) (45.1584, -3.4398) (45.0102, -3.3706) knots 0 0 0 1 2 2 2
  spline S449 degree 2 poles (45.0102, -3.3706) (44.8867, -3.3089) (44.5681, -3.2274) (44.3853, -3.2274) knots 0 0 0 1 2 2 2
  spline S450 degree 2 poles (44.3853, -3.2274) (43.9456, -3.2274) (43.4022, -3.8893) (43.4022, -4.4401) knots 0 0 0 1 2 2 2
  spline S451 degree 2 poles (43.4022, -4.4401) (43.4022, -4.7464) (43.5455, -5.2058) (43.6813, -5.3639) knots 0 0 0 1 2 2 2
  spline S452 degree 2 poles (43.6813, -5.3639) (43.8122, -5.522) (44.1827, -5.6875) (44.4149, -5.6875) knots 0 0 0 1 2 2 2
  spline S453 degree 2 poles (44.4149, -5.6875) (44.5853, -5.6875) (44.9262, -5.6381) (45.0423, -5.5887) knots 0 0 0 1 2 2 2
  line L427 (45.0423, -5.5887) -> (45.0423, -4.8008)
  line L428 (45.0423, -4.8008) -> (44.3359, -4.8008)
  line L429 (44.3359, -4.8008) -> (44.3359, -4.4451)
  line L430 (44.3359, -4.4451) -> (45.4424, -4.4451)
  line L431 (45.4424, -4.4451) -> (45.4424, -5.7764)
  spline S454 degree 2 poles (45.4424, -5.7764) (45.3659, -5.811) (45.104, -5.9172) (44.9929, -5.9493) knots 0 0 0 1 2 2 2
  spline S455 degree 2 poles (44.9929, -5.9493) (44.8422, -5.9938) (44.6002, -6.0382) (44.4297, -6.0382) knots 0 0 0 1 2 2 2
  spline S456 degree 2 poles (47.1961, -5.7369) (47.1492, -5.7715) (46.9911, -5.895) (46.917, -5.932) knots 0 0 0 1 2 2 2
  spline S457 degree 2 poles (46.917, -5.932) (46.8158, -5.9864) (46.6256, -6.0432) (46.4527, -6.0432) knots 0 0 0 1 2 2 2
  spline S458 degree 2 poles (46.4527, -6.0432) (46.3119, -6.0432) (46.0575, -5.937) (45.9611, -5.8406) knots 0 0 0 1 2 2 2
  spline S459 degree 2 poles (45.9611, -5.8406) (45.8698, -5.7468) (45.7586, -5.4701) (45.7586, -5.317) knots 0 0 0 1 2 2 2
  spline S460 degree 2 poles (45.7586, -5.317) (45.7586, -5.0799) (45.9587, -4.744) (46.176, -4.6476) knots 0 0 0 1 2 2 2
  spline S461 degree 2 poles (46.176, -4.6476) (46.3687, -4.5587) (46.8923, -4.492) (47.1961, -4.4747) knots 0 0 0 1 2 2 2
  line L432 (47.1961, -4.4747) -> (47.1961, -4.4006)
  spline S462 degree 2 poles (47.1961, -4.4006) (47.1961, -4.2672) (47.1146, -4.1017) (47.0405, -4.0548) knots 0 0 0 1 2 2 2
  spline S463 degree 2 poles (47.0405, -4.0548) (46.9664, -4.0079) (46.754, -3.9782) (46.6404, -3.9782) knots 0 0 0 1 2 2 2
  spline S464 degree 2 poles (46.6404, -3.9782) (46.507, -3.9782) (46.1464, -4.0573) (45.9661, -4.1339) knots 0 0 0 1 2 2 2
  line L433 (45.9661, -4.1339) -> (45.9439, -4.1339)
  line L434 (45.9439, -4.1339) -> (45.9439, -3.7411)
  spline S465 degree 2 poles (45.9439, -3.7411) (46.0501, -3.7115) (46.4477, -3.6374) (46.6429, -3.6374) knots 0 0 0 1 2 2 2
  spline S466 degree 2 poles (46.6429, -3.6374) (46.88, -3.6374) (47.2036, -3.7115) (47.332, -3.8078) knots 0 0 0 1 2 2 2
  spline S467 degree 2 poles (47.332, -3.8078) (47.458, -3.9017) (47.5815, -4.2005) (47.5815, -4.4154) knots 0 0 0 1 2 2 2
  line L435 (47.5815, -4.4154) -> (47.5815, -5.979)
  line L436 (47.5815, -5.979) -> (47.1961, -5.979)
  line L437 (47.1961, -5.979) -> (47.1961, -5.7369)
  line L438 (47.1961, -5.4158) -> (47.1961, -4.781)
  spline S468 degree 2 poles (47.1961, -4.781) (47.0578, -4.7934) (46.6404, -4.8353) (46.5095, -4.8749) knots 0 0 0 1 2 2 2
  spline S469 degree 2 poles (46.5095, -4.8749) (46.3563, -4.9218) (46.1563, -5.1169) (46.1563, -5.2898) knots 0 0 0 1 2 2 2
  spline S470 degree 2 poles (46.1563, -5.2898) (46.1563, -5.4874) (46.3786, -5.6875) (46.591, -5.6875) knots 0 0 0 1 2 2 2
  spline S471 degree 2 poles (46.591, -5.6875) (46.7713, -5.6875) (47.0677, -5.5319) (47.1961, -5.4158) knots 0 0 0 1 2 2 2
  spline S472 degree 2 poles (50.0391, -4.7983) (50.0391, -5.359) (49.4957, -6.0432) (49.0857, -6.0432) knots 0 0 0 1 2 2 2
  spline S473 degree 2 poles (49.0857, -6.0432) (48.9005, -6.0432) (48.6362, -5.9518) (48.5077, -5.8727) knots 0 0 0 1 2 2 2
  line L439 (48.5077, -5.8727) -> (48.483, -5.979)
  line L440 (48.483, -5.979) -> (48.1224, -5.979)
  line L441 (48.1224, -5.979) -> (48.1224, -2.7951)
  line L442 (48.1224, -2.7951) -> (48.5077, -2.7951)
  line L443 (48.5077, -2.7951) -> (48.5077, -3.9313)
  spline S474 degree 2 poles (48.5077, -3.9313) (48.6535, -3.8004) (48.9919, -3.6275) (49.2067, -3.6275) knots 0 0 0 1 2 2 2
  spline S475 degree 2 poles (49.2067, -3.6275) (49.5945, -3.6275) (50.0391, -4.2475) (50.0391, -4.7983) knots 0 0 0 1 2 2 2
  spline S476 degree 2 poles (49.6415, -4.8279) (49.6415, -4.4179) (49.392, -3.9931) (49.1154, -3.9931) knots 0 0 0 1 2 2 2
  spline S477 degree 2 poles (49.1154, -3.9931) (48.9597, -3.9931) (48.6386, -4.1413) (48.5077, -4.2549) knots 0 0 0 1 2 2 2
  line L444 (48.5077, -4.2549) -> (48.5077, -5.5665)
  spline S478 degree 2 poles (48.5077, -5.5665) (48.6535, -5.6381) (48.8782, -5.6974) (49.0116, -5.6974) knots 0 0 0 1 2 2 2
  spline S479 degree 2 poles (49.0116, -5.6974) (49.3055, -5.6974) (49.6415, -5.2799) (49.6415, -4.8279) knots 0 0 0 1 2 2 2
  line L445 (51.6521, -4.1042) -> (51.6323, -4.1042)
  spline S480 degree 2 poles (51.6323, -4.1042) (51.5878, -4.0919) (51.4915, -4.0869) (51.4248, -4.0869) knots 0 0 0 1 2 2 2
  spline S481 degree 2 poles (51.4248, -4.0869) (51.2692, -4.0869) (50.9629, -4.2228) (50.8246, -4.3562) knots 0 0 0 1 2 2 2
  line L446 (50.8246, -4.3562) -> (50.8246, -5.979)
  line L447 (50.8246, -5.979) -> (50.4393, -5.979)
  line L448 (50.4393, -5.979) -> (50.4393, -3.6917)
  line L449 (50.4393, -3.6917) -> (50.8246, -3.6917)
  line L450 (50.8246, -3.6917) -> (50.8246, -4.0326)
  spline S482 degree 2 poles (50.8246, -4.0326) (51.0346, -3.8449) (51.3482, -3.6917) (51.4964, -3.6917) knots 0 0 0 1 2 2 2
  spline S483 degree 2 poles (51.4964, -3.6917) (51.5557, -3.6917) (51.615, -3.6967) (51.6521, -3.7041) knots 0 0 0 1 2 2 2
  line L451 (51.6521, -3.7041) -> (51.6521, -4.1042)
  line L452 (52.3437, -5.979) -> (51.9583, -5.979)
  line L453 (51.9583, -5.979) -> (51.9583, -3.6917)
  line L454 (51.9583, -3.6917) -> (52.3437, -3.6917)
  line L455 (52.3437, -3.6917) -> (52.3437, -5.979)
  line L456 (52.3708, -3.3113) -> (51.9336, -3.3113)
  line L457 (51.9336, -3.3113) -> (51.9336, -2.9112)
  line L458 (51.9336, -2.9112) -> (52.3708, -2.9112)
  line L459 (52.3708, -2.9112) -> (52.3708, -3.3113)
  spline S484 degree 2 poles (53.9022, -6.0308) (53.3539, -6.0308) (52.7512, -5.4158) (52.7512, -4.8477) knots 0 0 0 1 2 2 2
  spline S485 degree 2 poles (52.7512, -4.8477) (52.7512, -4.2895) (53.3366, -3.6275) (53.8084, -3.6275) knots 0 0 0 1 2 2 2
  spline S486 degree 2 poles (53.8084, -3.6275) (54.0208, -3.6275) (54.3493, -3.751) (54.4703, -3.8819) knots 0 0 0 1 2 2 2
  spline S487 degree 2 poles (54.4703, -3.8819) (54.5938, -4.0128) (54.7248, -4.3907) (54.7248, -4.6649) knots 0 0 0 1 2 2 2
  line L460 (54.7248, -4.6649) -> (54.7248, -4.8749)
  line L461 (54.7248, -4.8749) -> (53.1415, -4.8749)
  spline S488 degree 2 poles (53.1415, -4.8749) (53.1415, -5.2725) (53.5416, -5.6949) (53.8973, -5.6949) knots 0 0 0 1 2 2 2
  spline S489 degree 2 poles (53.8973, -5.6949) (54.0233, -5.6949) (54.2678, -5.6381) (54.3666, -5.5936) knots 0 0 0 1 2 2 2
  spline S490 degree 2 poles (54.3666, -5.5936) (54.4703, -5.5442) (54.6136, -5.4578) (54.6605, -5.4183) knots 0 0 0 1 2 2 2
  line L462 (54.6605, -5.4183) -> (54.6828, -5.4183)
  line L463 (54.6828, -5.4183) -> (54.6828, -5.8382)
  spline S491 degree 2 poles (54.6828, -5.8382) (54.6161, -5.8653) (54.4135, -5.9444) (54.3345, -5.9666) knots 0 0 0 1 2 2 2
  spline S492 degree 2 poles (54.3345, -5.9666) (54.2233, -5.9987) (54.0406, -6.0308) (53.9022, -6.0308) knots 0 0 0 1 2 2 2
  spline S493 degree 2 poles (54.3493, -4.5809) (54.3444, -4.4253) (54.2802, -4.1981) (54.2184, -4.1215) knots 0 0 0 1 2 2 2
  spline S494 degree 2 poles (54.2184, -4.1215) (54.1517, -4.0351) (53.9418, -3.9437) (53.7862, -3.9437) knots 0 0 0 1 2 2 2
  spline S495 degree 2 poles (53.7862, -3.9437) (53.633, -3.9437) (53.4181, -4.0351) (53.3292, -4.124) knots 0 0 0 1 2 2 2
  spline S496 degree 2 poles (53.3292, -4.124) (53.2427, -4.2154) (53.1538, -4.4352) (53.1415, -4.5809) knots 0 0 0 1 2 2 2
  line L464 (53.1415, -4.5809) -> (54.3493, -4.5809)
  line L465 (55.5078, -5.979) -> (55.1224, -5.979)
  line L466 (55.1224, -5.979) -> (55.1224, -2.7951)
  line L467 (55.1224, -2.7951) -> (55.5078, -2.7951)
  line L468 (55.5078, -2.7951) -> (55.5078, -5.979)
  spline S497 degree 2 poles (57.0663, -6.0308) (56.518, -6.0308) (55.9153, -5.4158) (55.9153, -4.8477) knots 0 0 0 1 2 2 2
  spline S498 degree 2 poles (55.9153, -4.8477) (55.9153, -4.2895) (56.5007, -3.6275) (56.9725, -3.6275) knots 0 0 0 1 2 2 2
  spline S499 degree 2 poles (56.9725, -3.6275) (57.1849, -3.6275) (57.5134, -3.751) (57.6344, -3.8819) knots 0 0 0 1 2 2 2
  spline S500 degree 2 poles (57.6344, -3.8819) (57.7579, -4.0128) (57.8888, -4.3907) (57.8888, -4.6649) knots 0 0 0 1 2 2 2
  line L469 (57.8888, -4.6649) -> (57.8888, -4.8749)
  line L470 (57.8888, -4.8749) -> (56.3056, -4.8749)
  spline S501 degree 2 poles (56.3056, -4.8749) (56.3056, -5.2725) (56.7057, -5.6949) (57.0614, -5.6949) knots 0 0 0 1 2 2 2
  spline S502 degree 2 poles (57.0614, -5.6949) (57.1874, -5.6949) (57.4319, -5.6381) (57.5307, -5.5936) knots 0 0 0 1 2 2 2
  spline S503 degree 2 poles (57.5307, -5.5936) (57.6344, -5.5442) (57.7777, -5.4578) (57.8246, -5.4183) knots 0 0 0 1 2 2 2
  line L471 (57.8246, -5.4183) -> (57.8469, -5.4183)
  line L472 (57.8469, -5.4183) -> (57.8469, -5.8382)
  spline S504 degree 2 poles (57.8469, -5.8382) (57.7802, -5.8653) (57.5776, -5.9444) (57.4986, -5.9666) knots 0 0 0 1 2 2 2
  spline S505 degree 2 poles (57.4986, -5.9666) (57.3874, -5.9987) (57.2047, -6.0308) (57.0663, -6.0308) knots 0 0 0 1 2 2 2
  spline S506 degree 2 poles (57.5134, -4.5809) (57.5085, -4.4253) (57.4442, -4.1981) (57.3825, -4.1215) knots 0 0 0 1 2 2 2
  spline S507 degree 2 poles (57.3825, -4.1215) (57.3158, -4.0351) (57.1059, -3.9437) (56.9502, -3.9437) knots 0 0 0 1 2 2 2
  spline S508 degree 2 poles (56.9502, -3.9437) (56.7971, -3.9437) (56.5822, -4.0351) (56.4933, -4.124) knots 0 0 0 1 2 2 2
  spline S509 degree 2 poles (56.4933, -4.124) (56.4068, -4.2154) (56.3179, -4.4352) (56.3056, -4.5809) knots 0 0 0 1 2 2 2
  line L473 (56.3056, -4.5809) -> (57.5134, -4.5809)
  line L474 (-1.1, -36.8907) -> (1.5874, -36.8907)
  line L475 (1.5874, -36.8907) -> (1.5874, -35.8681)
  line L476 (1.5874, -35.8681) -> (1.948, -35.8681)
  line L477 (1.948, -35.8681) -> (1.948, -38.3184)
  line L478 (1.948, -38.3184) -> (1.5874, -38.3184)
  line L479 (1.5874, -38.3184) -> (1.5874, -37.2958)
  line L480 (1.5874, -37.2958) -> (-1.1, -37.2958)
  line L481 (-1.1, -37.2958) -> (-1.1, -36.8907)
  spline S510 degree 2 poles (0.0436, -40.4772) (-0.5344, -40.4772) (-1.1642, -39.9214) (-1.1642, -39.457) knots 0 0 0 1 2 2 2
  spline S511 degree 2 poles (-1.1642, -39.457) (-1.1642, -38.9803) (-0.5146, -38.4345) (0.0436, -38.4345) knots 0 0 0 1 2 2 2
  spline S512 degree 2 poles (0.0436, -38.4345) (0.6167, -38.4345) (1.2515, -38.9976) (1.2515, -39.457) knots 0 0 0 1 2 2 2
  spline S513 degree 2 poles (1.2515, -39.457) (1.2515, -39.9214) (0.6191, -40.4772) (0.0436, -40.4772) knots 0 0 0 1 2 2 2
  spline S514 degree 2 poles (0.0436, -40.0795) (0.4882, -40.0795) (0.9205, -39.7559) (0.9205, -39.457) knots 0 0 0 1 2 2 2
  spline S515 degree 2 poles (0.9205, -39.457) (0.9205, -39.1582) (0.4882, -38.8321) (0.0436, -38.8321) knots 0 0 0 1 2 2 2
  spline S516 degree 2 poles (0.0436, -38.8321) (-0.3886, -38.8321) (-0.8332, -39.1582) (-0.8332, -39.457) knots 0 0 0 1 2 2 2
  spline S517 degree 2 poles (-0.8332, -39.457) (-0.8332, -39.7534) (-0.396, -40.0795) (0.0436, -40.0795) knots 0 0 0 1 2 2 2
  line L482 (0.7747, -42.0851) -> (0.7747, -42.0654)
  spline S518 degree 2 poles (0.7747, -42.0654) (0.7871, -42.0209) (0.792, -41.9246) (0.792, -41.8579) knots 0 0 0 1 2 2 2
  spline S519 degree 2 poles (0.792, -41.8579) (0.792, -41.7023) (0.6562, -41.396) (0.5228, -41.2577) knots 0 0 0 1 2 2 2
  line L483 (0.5228, -41.2577) -> (-1.1, -41.2577)
  line L484 (-1.1, -41.2577) -> (-1.1, -40.8724)
  line L485 (-1.1, -40.8724) -> (1.1872, -40.8724)
  line L486 (1.1872, -40.8724) -> (1.1872, -41.2577)
  line L487 (1.1872, -41.2577) -> (0.8464, -41.2577)
  spline S520 degree 2 poles (0.8464, -41.2577) (1.0341, -41.4676) (1.1872, -41.7813) (1.1872, -41.9295) knots 0 0 0 1 2 2 2
  spline S521 degree 2 poles (1.1872, -41.9295) (1.1872, -41.9888) (1.1823, -42.0481) (1.1749, -42.0851) knots 0 0 0 1 2 2 2
  line L488 (1.1749, -42.0851) -> (0.7747, -42.0851)
  line L489 (1.948, -45.9334) -> (-1.1, -44.8837)
  line L490 (-1.1, -44.8837) -> (-1.1, -44.4465)
  line L491 (-1.1, -44.4465) -> (1.948, -43.3967)
  line L492 (1.948, -43.3967) -> (1.948, -43.8314)
  line L493 (1.948, -43.8314) -> (-0.5838, -44.6762)
  line L494 (-0.5838, -44.6762) -> (1.948, -45.5209)
  line L495 (1.948, -45.5209) -> (1.948, -45.9334)
  spline S522 degree 2 poles (-1.1519, -47.1882) (-1.1519, -46.6398) (-0.5368, -46.0372) (0.0313, -46.0372) knots 0 0 0 1 2 2 2
  spline S523 degree 2 poles (0.0313, -46.0372) (0.5895, -46.0372) (1.2515, -46.6226) (1.2515, -47.0943) knots 0 0 0 1 2 2 2
  spline S524 degree 2 poles (1.2515, -47.0943) (1.2515, -47.3067) (1.128, -47.6353) (0.997, -47.7563) knots 0 0 0 1 2 2 2
  spline S525 degree 2 poles (0.997, -47.7563) (0.8661, -47.8798) (0.4882, -48.0107) (0.2141, -48.0107) knots 0 0 0 1 2 2 2
  line L496 (0.2141, -48.0107) -> (0.0041, -48.0107)
  line L497 (0.0041, -48.0107) -> (0.0041, -46.4274)
  spline S526 degree 2 poles (0.0041, -46.4274) (-0.3936, -46.4274) (-0.8159, -46.8276) (-0.8159, -47.1832) knots 0 0 0 1 2 2 2
  spline S527 degree 2 poles (-0.8159, -47.1832) (-0.8159, -47.3092) (-0.7591, -47.5538) (-0.7147, -47.6526) knots 0 0 0 1 2 2 2
  spline S528 degree 2 poles (-0.7147, -47.6526) (-0.6653, -47.7563) (-0.5788, -47.8996) (-0.5393, -47.9465) knots 0 0 0 1 2 2 2